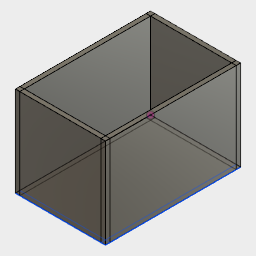
WiFiHousing v1 (Autodesk Fusion 360 design; units mm, degrees)
Autodesk Fusion 360 part; units mm, degrees
sketch "Sketch1" plane through (0, 0, 0) normal (0, 1, 0) x (1, 0, 0)
  line L0 (0, 0) -> (40, 0)
  line L1 (40, 0) -> (40, -60)
  line L2 (40, -60) -> (0, -60)
  line L3 (0, -60) -> (0, 0)
  line L4 (0, 0) -> (2, 0)
  line L5 (2, 0) -> (2, -60)
  line L6 (2, -60) -> (0, -60)
  line L7 (0, -60) -> (0, 0)
  line L8 (40, 0) -> (38, 0)
  line L9 (38, 0) -> (38, -60)
  line L10 (38, -60) -> (40, -60)
  line L11 (40, -60) -> (40, 0)
  line L12 (40, 0) -> (0, 0)
  line L13 (0, 0) -> (0, -2)
  line L14 (0, -2) -> (40, -2)
  line L15 (40, -2) -> (40, 0)
  line L16 (0, -60) -> (40, -60)
  line L17 (40, -60) -> (40, -58)
  line L18 (40, -58) -> (0, -58)
  line L19 (0, -58) -> (0, -60)
  dimension "d1" = 2
  dimension "d2" = 2
  dimension "d3" = 2
  dimension "d4" = 2
  measures "d1" distance of L0.start L4.end
  measures "d2" distance of L0.end L8.end
  measures "d3" distance of L0.end L14.end
  measures "d4" distance of L2.end L18.end
extrude "Extrude1" add sketch "Sketch1" along normal blind 40 contours L0 L5 L9 L12 L14 makes body 1
extrude "Extrude2" add sketch "Sketch1" along normal blind 40 separate body contours L3 L5 L7 L14 L18 makes body 2
extrude "Extrude3" add sketch "Sketch1" along normal blind 40 separate body contours L1 L9 L11 L14 L18 makes body 3
extrude "Extrude4" add sketch "Sketch1" along normal blind 40 separate body contours L2 L5 L9 L16 L18 makes body 4
extrude "Extrude5" add sketch "Sketch1" along normal blind 3 contours L5 L9 L14 L18 bodies 1 2 3 4
extrude "Extrude6" add sketch "Sketch1" along normal blind 40 separate body contours L0 L3 L4 L5 L7 L12 L13 L14 makes body 5
extrude "Extrude7" add sketch "Sketch1" along normal blind 40 separate body contours L2 L3 L5 L6 L7 L16 L18 L19 makes body 6
extrude "Extrude8" add sketch "Sketch1" along normal blind 40 separate body contours L1 L2 L9 L10 L11 L16 L17 L18 makes body 7
extrude "Extrude9" add sketch "Sketch1" along normal blind 40 separate body contours L0 L1 L8 L9 L11 L12 L14 L15 makes body 8
